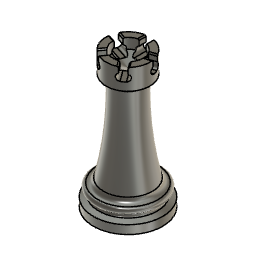
Rook (Autodesk Fusion 360 design; units mm, degrees)
Autodesk Fusion 360 part; units mm, degrees
note: some values were not read from the file. Set by a fixed rule: which sketch regions a step uses.
sketch "Szkic1" plane through (0, 0, 0) normal (0, 1, 0) x (1, 0, 0)
  line L0 (13, -5.5) -> (13, -16.9401) construction
  line L1 (0, 0) -> (15, 0)
  arc A0 (10.5635, -10.9401) -> (13, -9) centre (13, -11.5) cw
  line L2 (15, 0) -> (15, -3.7)
  line L3 (13, -5.5) -> (13, 0) construction
  line L4 (15, -3.7) -> (12.6552, -4.5613)
  arc A1 (13, -6.5) -> (13, -9) centre (13, -7.75) cw
  line L5 (0, 0) -> (13, 0) construction
  line L6 (0, -47.5) -> (0, -50)
  arc A2 (13, -6.5) -> (12.6552, -4.5613) centre (13, -5.5) cw
  line L7 (0, 0) -> (0, -59)
  line L8 (9.5, -59) -> (9.5, -50)
  line L9 (9.5, -50) -> (8.9268, -50)
  arc A3 (13.3263, -8.9567) -> (13, -9.5339) centre (67.7435, -40.0992) ccw
  arc A4 (10.5635, -10.9401) -> (6.9277, -48.0612) centre (152.678, -43.598) ccw
  arc A5 (6.9277, -48.0612) -> (8.9268, -50) centre (8.9268, -48) ccw
  line L10 (9.5, -59) -> (6.5, -59)
  line L11 (6.5, -59) -> (6.5, -54.5494)
  line L12 (6.5, -54.5494) -> (0, -52.1836)
  line L13 (6.5, -54.5494) -> (15.2621, -54.5494) construction
  point P0 (7, -50)
  dimension "d1" = 15
  dimension "d2" = 3.7
  dimension "d4" = 2
  dimension "d5" = 2.5
  dimension "d6" = 13
  dimension "d8" = 5
  dimension "d17" = 59
  dimension "d18" = 9.5
  dimension "d19" = 9
  dimension "d22" = 2.5
  dimension "d23" = 2
  dimension "d24" = 3
  dimension "d25" = 160
  constraint coincident L1.start L5.start
  constraint perpendicular L1 L2
  constraint tangent L4 A2
  constraint tangent A1 A2
  constraint coincident L3.end L1
  constraint coincident L0.start L3.start
  constraint parallel L0 L3
  constraint coincident A0.centre L0
  constraint coincident A1.centre L0
  constraint tangent A0 A1
  constraint perpendicular L1 L7
  constraint perpendicular L8 L9
  constraint coincident L0 A3.end
  constraint coincident A1 A3.start
  constraint tangent A0 A4
  constraint coincident P0 L9
  constraint coincident P0 A4
  constraint tangent L9 A5
  constraint tangent A4 A5
  constraint perpendicular L8 L10
  constraint perpendicular L10 L11
  constraint horizontal L13
  constraint coincident L7 L12.end
  measures "d1" distance of L1.end L1.start
  measures "d2" distance of L2.end L1.end
  measures "d4" diameter of A2
  measures "d5" diameter of A1
  measures "d6" distance of L3.end L1.start
  measures "d8" diameter of A0
  measures "d17" distance of L1.start L7.end
  measures "d18" distance of L7.end L8.start
  measures "d19" distance of L8.start L8.end
  measures "d22" distance of L8.end P0
  measures "d23" radius of A5
  measures "d24" distance of L8.start L10.end
  measures "d25" angle of L12 L13
revolve "Obrót1" add sketch "Szkic1" angle 360 about axis through (0, 0, 0) along (0, 0, 1)
sketch "Szkic3" plane through (0, 0, 0) normal (0, 1, 0) x (1, 0, 0)
  line L0 (1.5, -58.5) -> (1.5, -55.8725)
  line L1 (1, -55) -> (1, -53.5)
  line L2 (0, -64) -> (0, -51.6103)
  line L3 (1.5, -58.5) -> (3.6761, -60.6761)
  line L4 (1.5, -58.5) -> (3.7472, -58.5) construction
  line L5 (3.6761, -60.6761) -> (0, -60.6761)
  arc A0 (1.5, -56.4142) -> (1, -53.5) centre (1, -55) ccw
  line L6 (1, -53.5) -> (0, -53.5)
  line L7 (-3.6761, -60.6761) -> (0, -60.6761)
  line L8 (-1.5, -58.5) -> (-3.6761, -60.6761)
  line L9 (-1.5, -58.5) -> (-1.5, -55.8725)
  arc A1 (-1, -53.5) -> (-1.5, -56.4142) centre (-1, -55) ccw
  line L10 (-1, -53.5) -> (0, -53.5)
  line L11 (2.3, -59) -> (3.1, -59)
  line L12 (1.5, -58.5) -> (2.7, -58.5)
  line L13 (2.7, -58.5) -> (2.7, -59)
  dimension "d36" = 3
  dimension "d39" = 45
  constraint coincident L1.start A0.centre
  constraint vertical L1
  constraint vertical L2
  constraint horizontal L4
  constraint coincident L2 L5.end
  constraint perpendicular L2 L5
  constraint vertical L0
  constraint coincident L0 A0.start
  constraint coincident L2 L6.end
  constraint tangent A0 L6
  constraint symmetric L0.end L2 L9.end
  constraint symmetric L1.end L2 A1.start
  constraint symmetric L2 L0.start L8.start
  constraint symmetric L2 L3.end L7.start
  constraint symmetric L2 L5.end L7.end
  constraint symmetric L2 A0.start A1.end
  constraint symmetric L2 A0 A1
  constraint symmetric L2 L6.end L10.end
  constraint parallel L7 L11
  constraint coincident L4 L12.end
  constraint perpendicular L0 L12
  constraint midpoint L11 L13.end
  constraint perpendicular L11 L13
  measures "d36" diameter of A0
  measures "d39" angle of L3 L4
extrude "Wyciągnięcie proste2" cut sketch "Szkic3" along normal blind 14
pattern_circular "Szyk kołowy2" count 5 over 360 about axis through (0, 0, 1.75) along (0, 0, 1) of "Wyciągnięcie proste2"
